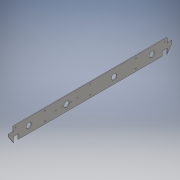
# Autodesk Inventor part: InsidePlate
Saved by Autodesk Inventor 2016 (Build 200138000, 138)
## iProperties
Created: 2017-01-13
Part Number: InsidePlate
Material: Generic
Document SubType Name: Modeling
Designer: hamblettk
Density: 1 g/cm^3
Appearance: Default
Author: hamblettk
Autodesk Inventor part; units mm, degrees
ref_plane "YZ Plane" through (0, 0, 0) normal (1, 0, 0) x (0, 1, 0)
ref_plane "XZ Plane" through (0, 0, 0) normal (0, 1, 0) x (-1, 0, 0)
ref_plane "XY Plane" through (0, 0, 0) normal (0, 0, 1) x (1, 0, 0)
sketch "Sketch1" plane through (0, 0, 0) normal (1, 0, 0) x (0, 1, 0)
  line L0 (0, 0) -> (76.2, 0)
  line L1 (76.2, 0) -> (76.2, -863.6)
  line L2 (76.2, -863.6) -> (0, -863.6)
  line L3 (0, -863.6) -> (0, 0)
  dimension "d0" = 76.2
  dimension "d1" = 863.6
  constraints: 8 end point, 2 parallel, 1 horizontal, 1 perpendicular
  measures "d0" distance of L1.end L2.end
  measures "d1" distance of L0.end L1.end
extrude "Extrusion1" add sketch "Sketch1" along normal blind 3.175
sketch "Sketch2" plane through (3.175, 0, 0) normal (1, 0, 0) x (0, 0, -1)
  line L0 (0, 38.1) -> (0, 36.5125)
  line L1 (0, 36.5125) -> (0, 39.6875)
  circle A0 centre (306.07, 36.5125) radius 14.2875
  circle A1 centre (557.53, 36.5125) radius 14.2875
  circle A2 centre (105.4351, 39.6875) radius 14.2875
  circle A3 centre (758.1649, 39.6875) radius 14.2875
  line L2 (863.6, 0) -> (838.2, 0)
  line L3 (863.6, 0) -> (863.6, 38.1)
  line L4 (863.6, 38.1) -> (838.2, 0)
  circle A4 centre (12.7, 63.5) radius 3.175
  line L5 (863.6, 76.2) -> (0, 76.2) projected
  circle A5 centre (850.9, 63.5) radius 3.175
  circle A6 centre (825.5, 15.875) radius 3.175
  circle A7 centre (38.1, 15.875) radius 3.175
  circle A8 centre (190.5, 15.875) radius 3.175
  circle A9 centre (431.8, 15.875) radius 3.175
  circle A10 centre (431.8, 63.5) radius 3.175
  circle A11 centre (673.1, 63.5) radius 3.175
  circle A12 centre (673.1, 15.875) radius 3.175
  circle A13 centre (190.5, 63.5) radius 3.175
  line L6 (0, 0) -> (25.4, 0)
  line L7 (0, 0) -> (0, 38.1)
  line L8 (0, 38.1) -> (25.4, 0)
  line L9 (863.6, 0) -> (0, 0) projected
  dimension "d15" = 28.575
  dimension "d16" = 28.575
  dimension "d19" = 28.575
  dimension "d21" = 28.575
  dimension "d22" = 25.4
  dimension "d26" = 6.35
  dimension "d27" = 12.7
  dimension "d29" = 6.35
  dimension "d30" = 12.7
  dimension "d32" = 6.35
  dimension "d34" = 12.7
  dimension "d35" = 6.35
  dimension "d39" = 6.35
  dimension "d40" = 863.6
  dimension "d41" = 6.35
  dimension "d43" = 6.35
  dimension "d44" = 12.7
  dimension "d45" = 6.35
  dimension "d46" = 6.35
  dimension "d48" = 241.3
  dimension "d49" = 241.3
  dimension "d50" = 6.35
  dimension "d51" = 241.3
  dimension "d53" = 241.3
  dimension "d54" = 25.4
  dimension "d55" = 38.1
  dimension "d58" = 15.875
  dimension "d59" = 15.875
  dimension "d60" = 15.875
  constraints: 16 end point, 14 centre point, 1 vertical
  measures "d15" diameter of A0
  measures "d16" diameter of A1
  measures "d19" diameter of A2
  measures "d21" diameter of A3
  measures "d22" distance of L2.start L2.end
  measures "d26" diameter of A4
  measures "d27" distance from line of L5 A4.centre
  measures "d29" diameter of A5
  measures "d30" distance from line of L5 A5.centre
  measures "d32" diameter of A6
  measures "d34" horizontal distance of L2.end A6.centre
  measures "d35" diameter of A7
  measures "d39" diameter of A8
  measures "d40" distance of L5.start L5.end
  measures "d41" diameter of A9
  measures "d43" diameter of A10
  measures "d44" distance from line of L5 A10.centre
  measures "d45" diameter of A11
  measures "d46" diameter of A12
  measures "d48" distance of A10.centre A11.centre
  measures "d49" distance of A12.centre A9.centre
  measures "d50" diameter of A13
  measures "d51" distance of A10.centre A13.centre
  measures "d53" distance of A9.centre A8.centre
  measures "d54" distance of L6.start L6.end
  measures "d55" distance of L6.start L0.start
  measures "d58" distance from line of L9 A8.centre
  measures "d59" distance from line of L9 A9.centre
  measures "d60" distance from line of L9 A12.centre
extrude "Extrusion3" cut sketch "Sketch2" against normal blind 25.4
sketch "Sketch3" plane through (3.175, 0, 0) normal (1, 0, 0) x (0, 0, -1)
  line L0 (0, 76.2) -> (863.6, 76.2) projected
  line L1 (0, 76.2) -> (25.4, 76.2)
  line L2 (25.4, 76.2) -> (25.4, 50.8)
  line L3 (25.4, 50.8) -> (0, 50.8)
  line L4 (0, 50.8) -> (0, 76.2)
  line L5 (25.4, 0) -> (50.8, 0)
  line L6 (50.8, 0) -> (50.8, 28.575)
  line L7 (50.8, 28.575) -> (25.4, 28.575)
  line L8 (25.4, 28.575) -> (25.4, 0)
  line L9 (863.6, 76.2) -> (838.2, 76.2)
  line L10 (838.2, 76.2) -> (838.2, 50.8)
  line L11 (838.2, 50.8) -> (863.6, 50.8)
  line L12 (863.6, 50.8) -> (863.6, 76.2)
  line L13 (50.8, 0) -> (812.8, 0)
  line L14 (812.8, 0) -> (812.8, 3.175)
  line L15 (812.8, 3.175) -> (50.8, 3.175)
  line L16 (50.8, 3.175) -> (50.8, 0)
  line L17 (838.2, 0) -> (812.8, 0)
  line L18 (812.8, 0) -> (812.8, 28.575)
  line L19 (812.8, 28.575) -> (838.2, 28.575)
  line L20 (838.2, 28.575) -> (838.2, 0)
  circle A0 centre (38.1, 63.5) radius 3.175
  circle A1 centre (825.5, 63.5) radius 3.175
  circle A2 centre (306.07, 36.5125) radius 14.2875 projected
  circle A3 centre (329.8825, 36.5125) radius 2.413
  circle A4 centre (363.22, 36.5125) radius 2.413
  circle A5 centre (282.2575, 36.5125) radius 2.413
  circle A6 centre (248.92, 36.5125) radius 2.413
  point P0 (0, 0)
  dimension "d63" = 25.4
  dimension "d64" = 25.4
  dimension "d65" = 25.4
  dimension "d66" = 28.575
  dimension "d67" = 25.4
  dimension "d68" = 25.4
  dimension "d77" = 762
  dimension "d78" = 3.175
  dimension "d79" = 25.4
  dimension "d80" = 28.575
  dimension "d81" = 6.35
  dimension "d82" = 6.35
  dimension "d88" = 4.826
  dimension "d89" = 4.826
  dimension "d90" = 4.826
  dimension "d91" = 4.826
  constraints: 40 end point, 10 parallel, 6 centre point, 5 horizontal, 5 perpendicular, 1 point on line
  measures "d63" distance of L2.end L3.end
  measures "d64" distance of L1.end L2.end
  measures "d65" distance of L7.end L6.end
  measures "d66" distance of L6.end L5.end
  measures "d67" distance of L11.end L10.end
  measures "d68" distance of L10.end L9.end
  measures "d77" distance of L15.end L14.end
  measures "d78" distance of L14.end L13.end
  measures "d79" distance of L18.end L19.end
  measures "d80" distance of L17.end L18.end
  measures "d81" diameter of A0
  measures "d82" diameter of A1
  measures "d88" diameter of A3
  measures "d89" diameter of A4
  measures "d90" diameter of A5
  measures "d91" diameter of A6
extrude "Extrusion5" cut sketch "Sketch3" against normal blind 25.4 contours L0 L12 L11 L10 | L0 L2 L3 L4 | L8 L7 L6 L5 | L6 L15 L14 L13 | L14 L18 L19 L20 L17 | A0 | A1 | A3 | A4 | A5 | A6
body "Solid1"
